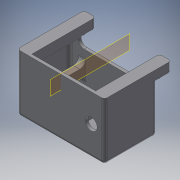
# Autodesk Inventor part: switchcase
Saved by Autodesk Inventor 2018 (Build 220112000, 112)
## iProperties
Created: 2017-12-11
Part Number: switchcase
Material: Generic
Document SubType Name: Modeling
Designer: ragna
Density: 1 g/cm^3
Appearance: Default
Author: ragna
Autodesk Inventor part; units mm, degrees
ref_plane "YZ Plane" through (0, 0, 0) normal (1, 0, 0) x (0, 1, 0)
ref_plane "XZ Plane" through (0, 0, 0) normal (0, 1, 0) x (-1, 0, 0)
ref_plane "XY Plane" through (0, 0, 0) normal (0, 0, 1) x (1, 0, 0)
sketch "Sketch1" plane through (0, 0, 0) normal (0, 0, 1) x (1, 0, 0)
  line L0 (0, 90) -> (0, 0) projected
  line L1 (-8, 0) -> (-8, 90) projected
  line L2 (0, 10) -> (-8, 10)
  line L3 (-8, 10) -> (-8, -36)
  line L4 (-8, -36) -> (0, -36)
  line L5 (0, -36) -> (0, 10)
  line L6 (0, 0) -> (-8, 0)
  dimension "d0" = 46
  dimension "d21" = 10
  constraints: 10 end point, 2 horizontal, 2 parallel, 2 point on line, 1 perpendicular, 2 other
  measures "d0" distance of L3.end L2.end
  measures "d21" distance between parallel lines of L6 L2
ref_plane "Work Plane1" through (-10.5787, -0.1763, 7) normal (0, 0, 1) x (1, 0, 0)
extrude "Extrusion1" add sketch "Sketch1" along normal up to surface (7 mm away)
sketch "Sketch2" plane through (0, 0, 0) normal (0, 0, -1) x (-1, 0, 0)
  circle A0 centre (4, 4.5) radius 1.5 projected
  point P0 (0, 0)
ref_plane "Work Plane2" through (-11.3807, -1.2929, -2) normal (0, 0, -1) x (0, 1, 0)
extrude "Extrusion2" add sketch "Sketch2" along normal up to surface (2 mm away)
ref_plane "Work Plane3" through (22, 90, -2) normal (1, 0, 0) x (0, 0, -1)
mirror "Mirror1" about plane through (22, 90, -2) normal (1, 0, 0)
sketch "Sketch3" plane through (0, -36, 0) normal (1, 0, 0) x (0, 0, -1)
  line L0 (0, 0) -> (-7, 0) projected
  line L1 (-7, 46) -> (-7, 0) projected
  line L2 (0, 0) -> (-7, 0)
  line L3 (-7, 0) -> (-7, 2)
  line L4 (-7, 2) -> (0, 2)
  line L5 (0, 2) -> (0, 0)
  point P0 (0, 36)
  dimension "d5" = 2
  constraints: 8 end point, 2 parallel, 1 horizontal, 1 perpendicular, 1 point on line
  measures "d5" distance of L2.end L3.end
extrude "Extrusion3" add sketch "Sketch3" along normal up to surface (44 mm away)
sketch "Sketch4" plane through (0, 0, 0) normal (0, 0, -1) x (-1, 0, 0)
  line L0 (-1.5, 0) -> (9.5, 0) projected
  line L1 (-53.5, 0) -> (-42.5, 0) projected
  circle A0 centre (-48, 4.5) radius 1.5 projected
  circle A1 centre (4, 4.5) radius 1.5 projected
  line L2 (0, 10) -> (8, 10) projected
  line L3 (0, -34) -> (0, 10) projected
  line L4 (0, -34) -> (-44, -34) projected
  line L5 (-44, -34) -> (-44, 10) projected
  line L6 (-44, 10) -> (-52, 10) projected
  line L7 (-52, 10) -> (-52, -36) projected
  line L8 (8, -36) -> (-52, -36) projected
  line L9 (8, 10) -> (8, -36) projected
  line L10 (8, -36) -> (8, 10) projected
  line L11 (8, -36) -> (-52, -36) projected
  line L12 (8, 0) -> (6, 0)
  line L13 (6, 0) -> (6, -36)
  line L14 (6, -36) -> (8, -36)
  line L15 (8, -36) -> (8, 0)
  line L16 (-52, -36) -> (-52, 10) projected
  line L17 (8, -36) -> (-52, -36) projected
  line L18 (-52, 0) -> (-50, 0)
  line L19 (-50, 0) -> (-50, -36)
  line L20 (-50, -36) -> (-52, -36)
  line L21 (-52, -36) -> (-52, 0)
  line L22 (6, -36) -> (-50, -36)
  line L23 (-50, -36) -> (-50, -34)
  line L24 (-50, -34) -> (6, -34)
  line L25 (6, -34) -> (6, -36)
  point P0 (0, 0)
  dimension "d8" = 2
  dimension "d9" = 2
  constraints: 24 end point, 7 point on line, 6 parallel, 3 horizontal, 3 perpendicular
  measures "d8" distance of L14.end L13.end
  measures "d9" distance of L19.end L20.end
ref_plane "Work Plane4" through (3.9425, -31.0984, -29.4) normal (0, 0, -1) x (0, 1, 0)
extrude "Extrusion4" add sketch "Sketch4" along normal up to surface (29.4 mm away) contours L0 L9 L8 L13 | L13 L8 L19 L24 L4 | L8 L7 L1 L19
sketch "Sketch5" plane through (0, 0, 0) normal (0, 0, -1) x (-1, 0, 0)
  line L0 (-52, 0) -> (-50, 0) projected
  line L1 (6, -34) -> (6, 0) projected
  line L2 (-50, 0) -> (6, 0)
  line L3 (6, 0) -> (6, -2)
  line L4 (6, -2) -> (-50, -2)
  line L5 (-50, -2) -> (-50, 0)
  point P0 (0, 0)
  dimension "d12" = 2
  constraints: 8 end point, 2 parallel, 1 horizontal, 1 perpendicular, 1 point on line
  measures "d12" distance of L2.end L3.end
extrude "Extrusion5" add sketch "Sketch5" along normal up to surface (29.4 mm away)
sketch "Sketch6" plane through (-8, 0, -29.4) normal (0, 1, 0) x (1, 0, 0)
  line L0 (52, -29.4) -> (8, -29.4) projected
  line L1 (52, -29.4) -> (8, -29.4)
  line L2 (8, -29.4) -> (8, -25.4)
  line L3 (8, -25.4) -> (52, -25.4)
  line L4 (52, -25.4) -> (52, -29.4)
  dimension "d15" = 4
  constraints: 8 end point, 2 parallel, 1 horizontal, 1 perpendicular
  measures "d15" distance of L1.end L2.end
extrude "Extrusion6" cut sketch "Sketch6" against normal up to surface (2 mm away)
sketch "Sketch7" plane through (0, -34, 7) normal (0, 1, 0) x (1, 0, 0)
  circle A0 centre (42.9512, 19.1747) radius 4.1
  point P0 (0, 7)
  constraints: 1 centre point
extrude "Extrusion7" cut sketch "Sketch7" against normal blind 10
sketch "Sketch8" plane through (0, -34, 7) normal (0, 1, 0) x (1, 0, 0)
  line L0 (28, 20.45) -> (32.85, 20.45) projected
  line L1 (28, 36.4) -> (28, 20.45) projected
  line L2 (5.4, 20.45) -> (0.55, 20.45) projected
  line L3 (5.4, 36.4) -> (5.4, 20.45) projected
  line L4 (32.85, 20.45) -> (28.3, 20.45)
  line L5 (28.3, 20.45) -> (28.3, 26.45)
  line L6 (28.3, 26.45) -> (32.85, 26.45)
  line L7 (32.85, 26.45) -> (32.85, 20.45)
  line L8 (0.55, 20.45) -> (5.1, 20.45)
  line L9 (5.1, 20.45) -> (5.1, 26.45)
  line L10 (5.1, 26.45) -> (0.55, 26.45)
  line L11 (0.55, 26.45) -> (0.55, 20.45)
  point P0 (0, 7)
  dimension "d22" = 6
  dimension "d23" = 0.3
  dimension "d24" = 0.3
  constraints: 16 end point, 4 parallel, 2 horizontal, 2 perpendicular, 1 point on line
  measures "d22" distance of L4.end L5.end
  measures "d23" distance between parallel lines of L1 L5
  measures "d24" distance between parallel lines of L3 L9
extrude "Extrusion8" add sketch "Sketch8" along normal up to surface (32 mm away)
sketch "Sketch9" plane through (0.55, -34, -13.45) normal (0, 0, 1) x (1, 0, 0)
  circle A0 centre (2.25, 11.758) radius 1.05 projected
  circle A1 centre (30.05, 11.758) radius 1.05 projected
  point P0 (-0.55, 34)
extrude "Extrusion9" cut sketch "Sketch9" against normal through all
sketch "Sketch10" plane through (52, 0, -29.4) normal (0, 0, -1) x (-1, 0, 0)
  line L0 (0, 0) -> (60, 0) projected
  line L1 (0, -36) -> (0, 0) projected
  line L2 (60, -36) -> (0, -36) projected
  line L3 (60, 0) -> (60, -36) projected
  line L4 (58, -2) -> (2, -2) projected
  line L5 (58, -34) -> (58, -2) projected
  line L6 (2, -34) -> (58, -34) projected
  line L7 (2, -2) -> (2, -34) projected
  point P0 (52, 0)
extrude "Extrusion10" add sketch "Sketch10" along normal blind 1
sketch "Sketch11" plane through (52, 0, -30.4) normal (0, 0, -1) x (-1, 0, 0)
  line L0 (58, -2) -> (58, -34) projected
  line L1 (58, -34) -> (2, -34) projected
  line L2 (2, -34) -> (2, -2) projected
  line L3 (2, -2) -> (58, -2) projected
  line L4 (60, 0) -> (0, 0) projected
  line L5 (0, 0) -> (0, -36) projected
  line L6 (0, -36) -> (60, -36) projected
  line L7 (60, -36) -> (60, 0) projected
  point P0 (52, 0)
extrude "Extrusion11" add sketch "Sketch11" along normal blind 2 contours L0 L1 L2 L3 | L7 L6 L5 L4
fillet "Fillet1" radius 2 20 edges at (50, -2, -15.2) (52, 0, -16.2) (52, -36, -12.7) (50, -34, -15.2) (-6, -2, -15.2) (-6, -34, -15.2) (-8, 0, -16.2) (-8, -36, -12.7) (22, -36, -32.4) (52, -18, -32.4) (22, 0, -32.4) (-8, -18, -32.4) (22, -2, -30.4) (-6, -18, -30.4) (22, -34, -30.4) (50, -18, -30.4) (-8, 10, 3.5) (0, 10, 3.5) (52, 10, 3.5) (44, 10, 3.5)
fillet "Fillet1" radius 4 10 edges at (0, -1, -4) (44, -1, -4) (30.575, -34, -13.45) (30.575, -2, -13.45) (2.825, -2, -13.45) (2.825, -34, -13.45) (2.825, -34, -19.45) (30.575, -34, -19.45) (2.825, -2, -19.45) (30.575, -2, -19.45)
fillet "Fillet1" radius 1 6 edges at (0, 5, 0) (-8, 5, 0) (52, 5, 0) (44, 5, 0) (48, 10, 0) (-4, 10, 0)
equation "\"d24\" = d23"
body "Solid1"
